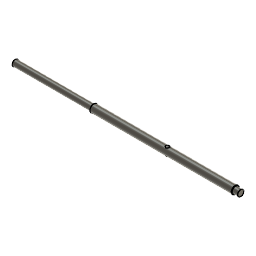
output-shaft (Autodesk Fusion 360 design; units mm, degrees)
part number: 2026-06-06-16-08-12-046
Autodesk Fusion 360 part; units mm, degrees
sketch "Sketch1" plane through (0, 0, 0) normal (1, 0, 0) x (0, 1, 0)
  circle A0 centre (0, 0) radius 5
  dimension "d1" = 10
  constraint coincident A0.centre origin
  measures "d1" diameter of A0
extrude "Extrude1" add sketch "Sketch1" along normal blind 180
sketch "Sketch2" plane through (180, 0, 0) normal (1, 0, 0) x (0, 1, 0)
  circle A0 centre (0, 0) radius 5
  circle A1 centre (0, 0) radius 4
  dimension "d4" = 8
  constraint coincident A0.centre A1.centre
  measures "d4" diameter of A1
extrude "Extrude2" cut sketch "Sketch2" against normal blind 20
sketch "Sketch3" plane through (0, 0, 0) normal (-1, 0, 0) x (0, -1, 0)
  circle A0 centre (0, 0) radius 5
  circle A1 centre (0, 0) radius 4
  dimension "d7" = 8
  constraint coincident A0.centre A1.centre
  measures "d7" diameter of A1
extrude "Extrude3" cut sketch "Sketch3" against normal blind 100
extrude "Extrude4" add 1 faces at (160, 4.6332, -0.4471) along direction (1, 0, 0) blind 5
extrude "Extrude5" cut 1 faces at (180, -1.2456, 0.0132) along direction (-1, 0, 0) blind 5
extrude "Extrude6" add 1 faces at (175, -1.2456, 0.0132) along direction (1, 0, 0) blind 26
extrude "Extrude7" add 1 faces at (165, 4.6332, -0.4471) along direction (1, 0, 0) blind 26
extrude "Extrude8" add 1 faces at (100, 4.6332, 0.4471) along direction (-1, 0, 0) blind 26
extrude "Extrude9" cut 1 faces at (0, 0.2111, 0.732) along direction (1, 0, 0) blind 30.1
extrude "Extrude10" add 1 faces at (30.1, 0.2111, 0.732) along direction (-1, 0, 0) blind 0.1
extrude "Extrude11" cut 1 faces at (30, 0.2111, 0.732) along direction (1, 0, 0) blind 1
extrude "Extrude12" add 1 faces at (31, 0.2111, 0.732) along direction (-1, 0, 0) blind 10
extrude "Extrude13" add 1 faces at (21, 0.2111, 0.732) along direction (-1, 0, 0) blind 10
sketch "Sketch4" plane through (0, 0, 0) normal (0, 0, 1) x (1, 0, 0)
  line L0 (191, 0) -> (186, 0)
  circle A0 centre (186, 0) radius 2.25
  circle A1 centre (161, 0) radius 2.25
  dimension "d30" = 5
  dimension "d31" = 4.5
  dimension "d35" = 4.5
  constraint horizontal L0
  constraint coincident L0.end A0.centre
  measures "d30" distance of L0.start L0.end
  measures "d31" diameter of A0
  measures "d35" diameter of A1
sketch "Sketch5" plane through (0, 0, 0) normal (0, 0, 1) x (1, 0, 0)
  circle A0 centre (161, 0) radius 2.25
  line L0 (191, -5) -> (191, 5)
  dimension "d38" = 4.5
  dimension "d39" = 30
  measures "d38" diameter of A0
  measures "d39" distance of A0.centre L0
extrude "Extrude17" add 1 faces at (11, 0.2111, 0.732) along direction (-1, 0, 0) blind 63
extrude "Extrude18" add 1 faces at (74, 4.6332, 0.4471) along direction (-1, 0, 0) blind 63
extrude "Extrude19" add 1 faces at (-52, 0.2111, 0.732) along direction (-1, 0, 0) blind 37
extrude "Extrude20" cut 1 faces at (201, -1.2456, 0.0132) along direction (-1, 0, 0) blind 3
sketch "Sketch6" plane through (0, 0, 0) normal (0, 0, 1) x (1, 0, 0)
  line L0 (190, 0) -> (105, 0)
  circle A0 centre (105, 0) radius 2.25
  dimension "d50" = 4.5
  constraint horizontal L0
  constraint coincident L0.end A0.centre
  measures "d50" diameter of A0
extrude "Extrude21" cut sketch "Sketch6" along normal mid plane 20
